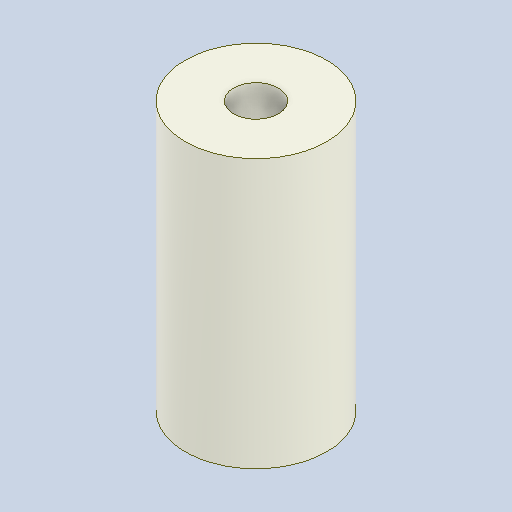
# Autodesk Inventor part: SMA-PanelMount-Ni-AuPlated-Dielectric
Saved by Autodesk Inventor 2026 (Build 300175050, 175E)
## iProperties
Created: 2026-02-17
Part Number: SMA-PanelMount-Ni-AuPlated-Dielectric
Material: Polytetrafluoroethylene
Document SubType Name: Modeling
Designer: schanen
Density: 2.02 g/cm^3
Appearance: Smooth - Ivory
Author: schanen
Autodesk Inventor part; units mm, degrees
ref_plane "YZ Plane" through (0, 0, 0) normal (1, 0, 0) x (0, 1, 0)
ref_plane "XZ Plane" through (0, 0, 0) normal (0, 1, 0) x (-1, 0, 0)
ref_plane "XY Plane" through (0, 0, 0) normal (0, 0, 1) x (1, 0, 0)
sketch "Sketch1" plane through (0, 0, 0) normal (0, 1, 0) x (-1, 0, 0)
  circle A0 centre (0, 0) radius 2
  circle A1 centre (0, 0) radius 0.635
  dimension "d0" = 4
  dimension "d1" = 1.27
  constraints: 2 centre point, 2 coincident
  measures "d0" diameter of A0
  measures "d1" diameter of A1
extrude "Extrusion1" add sketch "Sketch1" along normal blind 7.6
body "Solid1"
